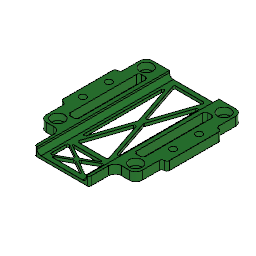
RM Carriage Setup (Goalie) (Autodesk Fusion 360 archive; units mm, degrees)
design "LGR RM Carriage Bracket (Goalie)"
Autodesk Fusion 360 part; units mm, degrees
(part 1 of 2)
sketch "Sketch1" plane through (0, 0, 0) normal (0, 0, 1) x (1, 0, 0)
  line L0 (-41, 41) -> (41, 41)
  line L1 (41, 41) -> (41, -41)
  line L2 (41, -41) -> (-41, -41)
  line L3 (-41, -41) -> (-41, 41)
  dimension "d1" = 82
  dimension "d2" = 82
  dimension "d3" = 41
  dimension "d4" = 41
  constraint horizontal L0
  constraint vertical L1
  constraint horizontal L2
  constraint vertical L3
  measures "d1" distance of L1 L3
  measures "d2" distance of L0 L2
  measures "d3" distance of origin L1
  measures "d4" distance of origin L0
extrude "Extrude1" add sketch "Sketch1" along normal blind 6.5
sketch "Sketch2" plane through (0, 0, 6.5) normal (0, 0, 1) x (-1, 0, 0)
  line L0 (41, 41) -> (-41, 41)
  line L1 (-41, 41) -> (-41, -41)
  line L2 (-41, -41) -> (41, -41)
  line L3 (41, -41) -> (41, 41)
  point P0 (34, -30)
  point P1 (-34, -30)
  point P2 (-34, 30)
  point P3 (34, 30)
  dimension "d7" = 68
  dimension "d8" = 60
  dimension "d9" = 7
  dimension "d10" = 11
  constraint horizontal P0 P1
  constraint vertical P1 P2
  constraint horizontal P2 P3
  constraint vertical P0 P3
  measures "d7" distance of P0 P1
  measures "d8" distance of P1 P2
  measures "d9" distance of L1 P1
  measures "d10" distance of L2 P1
hole "Hole1" at (-34, 30, 6.5) at (34, 30, 6.5) at (34, -30, 6.5) at (-34, -30, 6.5) direction (0, 0, -1) diameter 5.5 depth 10 tip angle 180 counterbore diameter 10 counterbore depth 5
sketch "Sketch3" plane through (0, 0, 6.5) normal (0, 0, 1) x (-1, 0, 0)
  circle A0 centre (-34, 30) radius 5
  circle A1 centre (34, -30) radius 5
  circle A2 centre (-34, -30) radius 5
  circle A3 centre (34, 30) radius 5
  line L0 (41, 41) -> (-41, 41)
  line L1 (-41, 41) -> (-41, -41)
  line L2 (-41, -41) -> (41, -41)
  line L3 (41, -41) -> (41, 41)
  line L4 (41, -19.05) -> (-41, -19.05)
  line L5 (-41, -19.05) -> (-41, 19.05)
  line L6 (-41, 19.05) -> (41, 19.05)
  line L7 (41, 19.05) -> (41, -19.05)
  dimension "d16" = 38.1
  dimension "d17" = 19.05
  constraint horizontal L4
  constraint vertical L5
  constraint horizontal L6
  constraint vertical L7
  constraint coincident L1 L5.end
  constraint coincident L3 L4.start
  measures "d16" distance of L4 L6
  measures "d17" distance of origin L6
extrude "Extrude2" cut sketch "Sketch3" against normal blind 4.5 contours L1 L3 L4 L5 L6 L7
fillet "Fillet1" radius 3 2 edges at (0, 19.05, 2) (0, -19.05, 2)
sketch "Sketch4" plane through (0, 0, 6.5) normal (0, 0, 1) x (-1, 0, 0)
  line L0 (41, -19.05) -> (-41, -19.05)
  line L1 (-41, -19.05) -> (-41, -41)
  line L2 (-41, -41) -> (41, -41)
  line L3 (41, -41) -> (41, -19.05)
  circle A0 centre (34, -30) radius 5
  circle A1 centre (-34, -30) radius 5
  line L4 (41, 41) -> (-41, 41)
  line L5 (41, 19.05) -> (41, 41)
  point P0 (-10, -34.75)
  point P1 (10, -34.75)
  point P2 (-10, 34.75)
  point P3 (10, 34.75)
  point P4 (-5.7919, 53.9874)
  dimension "d23" = 6.25
  dimension "d24" = 6.25
  dimension "d25" = 20
  dimension "d26" = 31
  constraint vertical P0 P2
  constraint horizontal P2 P3
  constraint vertical P1 P3
  constraint horizontal P0 P1
  measures "d23" distance of P2 L4
  measures "d24" distance of L2 P0
  measures "d25" distance of P0 P1
  measures "d26" distance of P3 L5
hole "Hole2" at (10, 34.75, 6.5) at (-10, 34.75, 6.5) at (10, -34.75, 6.5) at (-10, -34.75, 6.5) direction (0, 0, -1) diameter 5 end through all
sketch "Sketch7" plane through (0, 0, 6.5) normal (0, 0, 1) x (-1, 0, 0)
  circle A0 centre (-10, 34.75) radius 2.5
  circle A1 centre (10, 34.75) radius 2.5
  line L0 (-41, 19.05) -> (41, 19.05)
  line L1 (41, 19.05) -> (41, 41)
  line L2 (41, 41) -> (-41, 41)
  line L3 (-41, 41) -> (-41, 19.05)
  circle A2 centre (34, 30) radius 5
  circle A3 centre (-34, 30) radius 5
  line L4 (25.5, 22.05) -> (-25.5, 22.05)
  line L5 (-27.5, 24.05) -> (-27.5, 27.05)
  line L6 (-25.5, 29.05) -> (25.5, 29.05)
  line L7 (27.5, 27.05) -> (27.5, 24.05)
  line L8 (25.5, -29.05) -> (-25.5, -29.05)
  line L9 (-27.5, -27.05) -> (-27.5, -24.05)
  line L10 (-25.5, -22.05) -> (25.5, -22.05)
  line L11 (27.5, -24.05) -> (27.5, -27.05)
  line L12 (41, -19.05) -> (-41, -19.05)
  line L13 (-41, -19.05) -> (-41, -41)
  arc A4 (25.5, -29.05) -> (27.5, -27.05) centre (25.5, -27.05) ccw
  arc A5 (27.5, -24.05) -> (25.5, -22.05) centre (25.5, -24.05) ccw
  arc A6 (-25.5, -22.05) -> (-27.5, -24.05) centre (-25.5, -24.05) ccw
  arc A7 (-27.5, -27.05) -> (-25.5, -29.05) centre (-25.5, -27.05) ccw
  arc A8 (25.5, 22.05) -> (27.5, 24.05) centre (25.5, 24.05) ccw
  arc A9 (27.5, 27.05) -> (25.5, 29.05) centre (25.5, 27.05) ccw
  arc A10 (-25.5, 29.05) -> (-27.5, 27.05) centre (-25.5, 27.05) ccw
  arc A11 (-27.5, 24.05) -> (-25.5, 22.05) centre (-25.5, 24.05) ccw
  dimension "d31" = 55
  dimension "d32" = 7
  dimension "d33" = 3
  dimension "d34" = 13.5
  dimension "d35" = 7
  dimension "d36" = 3
  dimension "d37" = 13.5
  dimension "d38" = 55
  dimension "d39" = 2
  constraint horizontal L4
  constraint vertical L5
  constraint horizontal L6
  constraint vertical L7
  constraint horizontal L8
  constraint vertical L9
  constraint horizontal L10
  constraint vertical L11
  constraint tangent L8 A4
  constraint tangent L11 A4
  constraint tangent L11 A5
  constraint tangent L10 A5
  constraint equal A4 A5
  constraint tangent L10 A6
  constraint tangent L9 A6
  constraint equal A4 A6
  constraint tangent L9 A7
  constraint tangent L8 A7
  constraint equal A4 A7
  constraint tangent L4 A8
  constraint tangent L7 A8
  constraint equal A4 A8
  constraint tangent L7 A9
  constraint tangent L6 A9
  constraint equal A4 A9
  constraint tangent L6 A10
  constraint tangent L5 A10
  constraint equal A4 A10
  constraint tangent L5 A11
  constraint tangent L4 A11
  constraint equal A4 A11
  measures "d31" distance of L5 L7
  measures "d32" distance of L4 L6
  measures "d33" distance of L0 L4
  measures "d34" distance of L1 L7
  measures "d35" distance of L8 L10
  measures "d36" distance of L10 L12
  measures "d37" distance of L9 L13
  measures "d38" distance of L9 L11
  measures "d39" radius of A4
extrude "Extrude3" cut sketch "Sketch7" against normal blind 6.5 contours L4 L5 L6 L7 A8 A9 A10 A11 | L8 L9 L10 L11 A4 A5 A6 A7
ref_plane "WorkPlane1" through (0, 0, 6.5) normal (0, 0, -1) x (-1, 0, 0)
sketch "Sketch9" plane through (0, 0, 6.5) normal (0, 0, -1) x (-1, 0, 0)
  line L0 (41, 41) -> (21, 41)
  line L1 (21, 41) -> (21, 37)
  line L2 (21, 37) -> (41, 37)
  line L3 (41, 37) -> (41, 41)
  line L4 (-21, 41) -> (-41, 41)
  line L5 (-41, 41) -> (-41, 37)
  line L6 (-41, 37) -> (-21, 37)
  line L7 (-21, 37) -> (-21, 41)
  line L8 (41, -37) -> (21, -37)
  line L9 (21, -37) -> (21, -41)
  line L10 (21, -41) -> (41, -41)
  line L11 (41, -41) -> (41, -37)
  line L12 (-41, -41) -> (-21, -41)
  line L13 (-21, -41) -> (-21, -37)
  line L14 (-21, -37) -> (-41, -37)
  line L15 (-41, -37) -> (-41, -41)
  point P0 (41, 41)
  dimension "d59" = 82
  dimension "d60" = 82
  dimension "d61" = 4
  dimension "d62" = 20
  dimension "d63" = 20
  dimension "d64" = 4
  dimension "d65" = 20
  dimension "d66" = 20
  dimension "d67" = 4
  dimension "d68" = 4
  constraint horizontal L0
  constraint vertical L1
  constraint horizontal L2
  constraint vertical L3
  constraint horizontal L4
  constraint vertical L5
  constraint horizontal L6
  constraint vertical L7
  constraint horizontal L8
  constraint vertical L9
  constraint horizontal L10
  constraint vertical L11
  constraint horizontal L12
  constraint vertical L13
  constraint horizontal L14
  constraint vertical L15
  constraint vertical P0 L10.end
  constraint horizontal P0 L4.end
  constraint vertical L4.end L12.start
  constraint horizontal L10.end L12.start
  constraint vertical P0 L0.start
  constraint horizontal L0.end P0
  measures "d59" distance of L3 L5
  measures "d60" distance of L0 L10
  measures "d61" distance of L0 L2
  measures "d62" distance of L1 L3
  measures "d63" distance of L5 L7
  measures "d64" distance of L4 L6
  measures "d65" distance of L13 L15
  measures "d66" distance of L9 L11
  measures "d67" distance of L8 L10
  measures "d68" distance of L12 L14
extrude "Extrude5" cut sketch "Sketch9" along normal blind 6.5
fillet "Fillet2" radius 5 4 edges at (-41, 37, 3.25) (41, 37, 3.25) (41, -37, 3.25) (-41, -37, 3.25)
fillet "Fillet3" radius 2 8 edges at (-21, -41, 3.25) (-21, -37, 3.25) (21, -37, 3.25) (21, -41, 3.25) (21, 37, 3.25) (21, 41, 3.25) (-21, 41, 3.25) (-21, 37, 3.25)
sketch "Sketch10" plane through (0, 0, 2) normal (0, 0, 1) x (-1, 0, 0)
  line L0 (41, 16.05) -> (-41, 16.05)
  line L1 (-41, 16.05) -> (-41, -16.05)
  line L2 (-41, -16.05) -> (41, -16.05)
  line L3 (41, -16.05) -> (41, 16.05)
  line L4 (29.8377, -14) -> (-29.8377, -14)
  line L5 (29.8377, 14) -> (-29.8377, 14)
  line L6 (37.5, -10.6064) -> (37.5, 10.6064)
  line L7 (-37.5, -10.6064) -> (-37.5, 10.6064)
  line L8 (41, -19.05) -> (-41, -19.05)
  line L9 (30.154, 12.0513) -> (0.3162, 2.1054)
  line L10 (-0.3162, 2.1054) -> (-30.154, 12.0513)
  line L11 (-36.1798, 11.5537) -> (-4.8025, 0.9473)
  line L12 (-4.8025, -0.9473) -> (-36.1798, -11.5537)
  line L13 (-30.154, -12.0513) -> (-0.3162, -2.1054)
  line L14 (0.3162, -2.1054) -> (30.154, -12.0513)
  line L15 (36.1798, -11.5537) -> (4.8025, -0.9473)
  line L16 (4.8025, 0.9473) -> (36.1798, 11.5537)
  arc A0 (29.8377, -14) -> (30.154, -12.0513) centre (29.8377, -13) ccw
  arc A1 (0.3162, -2.1054) -> (-0.3162, -2.1054) centre (0, -3.0541) ccw
  arc A2 (-30.154, -12.0513) -> (-29.8377, -14) centre (-29.8377, -13) ccw
  arc A3 (-37.5, -10.6064) -> (-36.1798, -11.5537) centre (-36.5, -10.6064) ccw
  arc A4 (-36.1798, 11.5537) -> (-37.5, 10.6064) centre (-36.5, 10.6064) ccw
  arc A5 (-4.8025, -0.9473) -> (-4.8025, 0.9473) centre (-5.1228, 0) ccw
  arc A6 (-0.3162, 2.1054) -> (0.3162, 2.1054) centre (0, 3.0541) ccw
  arc A7 (-29.8377, 14) -> (-30.154, 12.0513) centre (-29.8377, 13) ccw
  arc A8 (30.154, 12.0513) -> (29.8377, 14) centre (29.8377, 13) ccw
  arc A9 (37.5, 10.6064) -> (36.1798, 11.5537) centre (36.5, 10.6064) ccw
  arc A10 (36.1798, -11.5537) -> (37.5, -10.6064) centre (36.5, -10.6064) ccw
  arc A11 (4.8025, 0.9473) -> (4.8025, -0.9473) centre (5.1228, 0) ccw
  point P0 (36, -14)
  point P1 (-36, -14)
  point P2 (-37.5, -12)
  point P3 (-37.5, 12)
  point P4 (0, -2)
  point P5 (-2, 0)
  point P6 (0, 2)
  point P7 (2, 0)
  dimension "d75" = 72
  dimension "d76" = 24
  dimension "d77" = 5
  dimension "d78" = 7.05
  dimension "d79" = 2.05
  dimension "d80" = 2.05
  dimension "d81" = 3.5
  dimension "d82" = 3.5
  dimension "d83" = 1
  constraint parallel L2 L4
  constraint perpendicular L3 L5
  constraint perpendicular L5 L6
  constraint perpendicular L4 L7
  constraint coincident P0 L4
  constraint coincident P0 L14
  constraint tangent L4 A0
  constraint tangent L14 A0
  constraint tangent L14 A1
  constraint tangent L13 A1
  constraint equal A0 A1
  constraint coincident P1 L13
  constraint coincident P1 L4
  constraint tangent L13 A2
  constraint tangent L4 A2
  constraint equal A0 A2
  constraint coincident P2 L12
  constraint coincident P2 L7
  constraint tangent L12 A3
  constraint tangent L7 A3
  constraint equal A0 A3
  constraint coincident P3 L7
  constraint coincident P3 L11
  constraint tangent L7 A4
  constraint tangent L11 A4
  constraint equal A0 A4
  constraint tangent L11 A5
  constraint tangent L12 A5
  constraint equal A0 A5
  constraint tangent L10 A6
  constraint tangent L9 A6
  constraint equal A0 A6
  constraint tangent L10 A7
  constraint tangent L5 A7
  constraint equal A0 A7
  constraint tangent L5 A8
  constraint tangent L9 A8
  constraint equal A0 A8
  constraint tangent L16 A9
  constraint tangent L6 A9
  constraint equal A0 A9
  constraint tangent L6 A10
  constraint tangent L15 A10
  constraint equal A0 A10
  constraint tangent L15 A11
  constraint tangent L16 A11
  constraint equal A0 A11
  measures "d75" distance of P0 P1
  measures "d76" distance of P2 P3
  measures "d77" distance of L1 P1
  measures "d78" distance of P2 L8
  measures "d79" distance of L2 L4
  measures "d80" distance of L0 L5
  measures "d81" distance of L1 L7
  measures "d82" distance of L3 L6
  measures "d83" radius of A0
extrude "Extrude6" cut sketch "Sketch10" against normal blind 2 contours L4 L13 L14 A0 A1 A2 | L5 L9 L10 A6 A7 A8 | L6 L15 L16 A9 A10 A11 | L7 L11 L12 A3 A4 A5
extrude "Extrude7" add 1 faces at (8.5, 16.6833, 0) along direction (0, 0, -1) blind 0.25
extrude "Extrude8" add 2 faces at (41, 10.6667, -0.0833) (41, 27.6732, 3.691) along direction (1, 0, 0) blind 20
sketch "Sketch12" plane through (0, 0, 6.5) normal (0, 0, 1) x (-1, 0, 0)
  arc A0 (-19, 41) -> (-21, 39) centre (-19, 39) ccw
  arc A1 (-23, 37) -> (-21, 39) centre (-23, 39) ccw
  line L0 (-23, 37) -> (-36, 37)
  arc A2 (-36, 37) -> (-41, 32) centre (-36, 32) ccw
  line L1 (-41, 32) -> (-61, 32)
  line L2 (-61, 32) -> (-61, 19.05)
  line L3 (-61, 19.05) -> (41, 19.05)
  line L4 (41, 19.05) -> (41, 32)
  arc A3 (41, 32) -> (36, 37) centre (36, 32) ccw
  line L5 (36, 37) -> (23, 37)
  arc A4 (21, 39) -> (23, 37) centre (23, 39) ccw
  arc A5 (21, 39) -> (19, 41) centre (19, 39) ccw
  line L6 (19, 41) -> (-19, 41)
  circle A6 centre (-34, 30) radius 5
  circle A7 centre (34, 30) radius 5
  circle A8 centre (10, 34.75) radius 2.5
  circle A9 centre (-10, 34.75) radius 2.5
  line L7 (-27.5, 24.05) -> (-27.5, 27.05)
  arc A10 (-25.5, 29.05) -> (-27.5, 27.05) centre (-25.5, 27.05) ccw
  line L8 (-25.5, 29.05) -> (25.5, 29.05)
  arc A11 (27.5, 27.05) -> (25.5, 29.05) centre (25.5, 27.05) ccw
  line L9 (27.5, 27.05) -> (27.5, 24.05)
  arc A12 (25.5, 22.05) -> (27.5, 24.05) centre (25.5, 24.05) ccw
  line L10 (25.5, 22.05) -> (-25.5, 22.05)
  arc A13 (-27.5, 24.05) -> (-25.5, 22.05) centre (-25.5, 24.05) ccw
  line L11 (-61, 32) -> (-41, 32)
  line L12 (-41, 32) -> (-41, 21.05)
  line L13 (-41, 21.05) -> (-61, 21.05)
  line L14 (-61, 21.05) -> (-61, 32)
  line L15 (-61, -32) -> (-41, -32)
  line L16 (-41, -32) -> (-41, -21.05)
  line L17 (-41, -21.05) -> (-61, -21.05)
  line L18 (-61, -21.05) -> (-61, -32)
  line L19 (41, -19.05) -> (-61, -19.05)
  dimension "d90" = 2
  dimension "d91" = 20
  dimension "d92" = 2
  dimension "d93" = 20
  dimension "d94" = 64
  constraint horizontal L11
  constraint vertical L12
  constraint horizontal L13
  constraint vertical L14
  constraint coincident L1.end L2.start
  constraint horizontal L15
  constraint vertical L16
  constraint horizontal L17
  constraint vertical L18
  constraint vertical L1.end L15.start
  measures "d90" distance of L3 L13
  measures "d91" distance of L12 L14
  measures "d92" distance of L17 L19
  measures "d93" distance of L16 L18
  measures "d94" distance of L11 L15
extrude "Extrude9" cut sketch "Sketch12" against normal blind 7 contours L1 L2 L11 L12 L13 L14 | L15 L16 L17 L18
fillet "Fillet4" radius 5 2 edges at (41, 21.05, 3.125) (41, -21.05, 3.125)
fillet "Fillet5" radius 1.5 2 edges at (61, 21.05, 3.125) (61, -21.05, 3.125)
sketch "Sketch14" plane through (0, 0, 2) normal (0, 0, 1) x (-1, 0, 0)
  line L0 (37.5, 10.6064) -> (37.5, -10.6064)
  arc A0 (36.1798, -11.5537) -> (37.5, -10.6064) centre (36.5, -10.6064) ccw
  line L1 (36.1798, -11.5537) -> (4.8025, -0.9473)
  arc A1 (4.8025, 0.9473) -> (4.8025, -0.9473) centre (5.1228, 0) ccw
  line L2 (4.8025, 0.9473) -> (36.1798, 11.5537)
  arc A2 (37.5, 10.6064) -> (36.1798, 11.5537) centre (36.5, 10.6064) ccw
  line L3 (30.154, 12.0513) -> (0.3162, 2.1054)
  arc A3 (-0.3162, 2.1054) -> (0.3162, 2.1054) centre (0, 3.0541) ccw
  line L4 (-0.3162, 2.1054) -> (-30.154, 12.0513)
  arc A4 (-29.8377, 14) -> (-30.154, 12.0513) centre (-29.8377, 13) ccw
  line L5 (-29.8377, 14) -> (29.8377, 14)
  arc A5 (30.154, 12.0513) -> (29.8377, 14) centre (29.8377, 13) ccw
  line L6 (-30.154, -12.0513) -> (-0.3162, -2.1054)
  arc A6 (0.3162, -2.1054) -> (-0.3162, -2.1054) centre (0, -3.0541) ccw
  line L7 (0.3162, -2.1054) -> (30.154, -12.0513)
  arc A7 (29.8377, -14) -> (30.154, -12.0513) centre (29.8377, -13) ccw
  line L8 (29.8377, -14) -> (-29.8377, -14)
  arc A8 (-30.154, -12.0513) -> (-29.8377, -14) centre (-29.8377, -13) ccw
  line L9 (-4.8025, -0.9473) -> (-36.1798, -11.5537)
  arc A9 (-37.5, -10.6064) -> (-36.1798, -11.5537) centre (-36.5, -10.6064) ccw
  line L10 (-37.5, -10.6064) -> (-37.5, 10.6064)
  arc A10 (-36.1798, 11.5537) -> (-37.5, 10.6064) centre (-36.5, 10.6064) ccw
  line L11 (-36.1798, 11.5537) -> (-4.8025, 0.9473)
  arc A11 (-4.8025, -0.9473) -> (-4.8025, 0.9473) centre (-5.1228, 0) ccw
  line L12 (41, 16.05) -> (-61, 16.05)
  line L13 (-61, 16.05) -> (-61, -16.05)
  line L14 (-61, -16.05) -> (41, -16.05)
  line L15 (41, -16.05) -> (41, 16.05)
  line L16 (-57.5, 10.5218) -> (-57.5, -10.5218)
  line L17 (-41, 10.5218) -> (-41, -10.5218)
  line L18 (-41.94, -10.7593) -> (-47.2368, -0.9503)
  line L19 (-47.2368, 0.9503) -> (-41.94, 10.7593)
  line L20 (-56.56, 10.7593) -> (-51.2632, 0.9503)
  line L21 (-51.2632, -0.9503) -> (-56.56, -10.7593)
  line L22 (-55.0268, 14) -> (-43.4732, 14)
  line L23 (-42.6049, 12.5039) -> (-48.3818, 2.3944)
  line L24 (-50.1182, 2.3944) -> (-55.8951, 12.5039)
  line L25 (-55.8951, -12.5039) -> (-50.1182, -2.3944)
  line L26 (-48.3818, -2.3944) -> (-42.6049, -12.5039)
  line L27 (-43.4732, -14) -> (-55.0268, -14)
  arc A12 (-55.0268, 14) -> (-55.8951, 12.5039) centre (-55.0268, 13) ccw
  arc A13 (-42.6049, 12.5039) -> (-43.4732, 14) centre (-43.4732, 13) ccw
  arc A14 (-55.8951, -12.5039) -> (-55.0268, -14) centre (-55.0268, -13) ccw
  arc A15 (-43.4732, -14) -> (-42.6049, -12.5039) centre (-43.4732, -13) ccw
  arc A16 (-48.3818, -2.3944) -> (-50.1182, -2.3944) centre (-49.25, -2.8906) ccw
  arc A17 (-50.1182, 2.3944) -> (-48.3818, 2.3944) centre (-49.25, 2.8906) ccw
  arc A18 (-41, 10.5218) -> (-41.94, 10.7593) centre (-41.5, 10.5218) ccw
  arc A19 (-41.94, -10.7593) -> (-41, -10.5218) centre (-41.5, -10.5218) ccw
  arc A20 (-57.5, -10.5218) -> (-56.56, -10.7593) centre (-57, -10.5218) ccw
  arc A21 (-51.2632, -0.9503) -> (-51.2632, 0.9503) centre (-53.023, 0) ccw
  arc A22 (-47.2368, 0.9503) -> (-47.2368, -0.9503) centre (-45.477, 0) ccw
  arc A23 (-56.56, 10.7593) -> (-57.5, 10.5218) centre (-57, 10.5218) ccw
  point P0 (-57.5, 12.5)
  point P1 (-57.5, -12.5)
  point P2 (-47.75, 0)
  point P3 (-50.75, 0)
  point P4 (-49.25, 0.875)
  point P5 (-56.75, -14)
  point P6 (-49.25, -0.875)
  point P7 (-41.75, -14)
  dimension "d106" = 3.5
  dimension "d107" = 3.5
  dimension "d108" = 2.05
  dimension "d109" = 2.05
  dimension "d110" = 25
  dimension "d111" = 12.5
  dimension "d112" = 15
  dimension "d113" = 0.75
  dimension "d114" = 3
  dimension "d115" = 1.75
  dimension "d116" = 1.5
  dimension "d117" = 0.875
  dimension "d118" = 8.25
  dimension "d119" = 1
  dimension "d120" = 0.5
  dimension "d121" = 2
  dimension "d122" = 0.5
  constraint vertical L16
  constraint perpendicular L12 L17
  constraint perpendicular L16 L22
  constraint horizontal P2 P3
  constraint vertical P4 P6
  constraint horizontal origin P2
  constraint tangent L24 A12
  constraint tangent L22 A12
  constraint tangent L22 A13
  constraint tangent L23 A13
  constraint equal A12 A13
  constraint coincident P5 L25
  constraint coincident P5 L27
  constraint tangent L25 A14
  constraint tangent L27 A14
  constraint equal A12 A14
  constraint coincident P7 L27
  constraint coincident P7 L26
  constraint tangent L27 A15
  constraint tangent L26 A15
  constraint equal A12 A15
  constraint coincident P6 L26
  constraint coincident P6 L25
  constraint tangent L26 A16
  constraint tangent L25 A16
  constraint equal A12 A16
  constraint coincident P4 L24
  constraint coincident P4 L23
  constraint tangent L24 A17
  constraint tangent L23 A17
  constraint equal A12 A17
  constraint tangent L19 A18
  constraint tangent L17 A18
  constraint tangent L17 A19
  constraint tangent L18 A19
  constraint equal A18 A19
  constraint coincident P1 L21
  constraint coincident P1 L16
  constraint tangent L21 A20
  constraint tangent L16 A20
  constraint equal A18 A20
  constraint coincident P3 L20
  constraint coincident P3 L21
  constraint tangent L20 A21
  constraint tangent L21 A21
  constraint coincident P2 L18
  constraint coincident P2 L19
  constraint tangent L18 A22
  constraint tangent L19 A22
  constraint equal A21 A22
  constraint coincident P0 L16
  constraint coincident P0 L20
  constraint tangent L16 A23
  constraint tangent L20 A23
  measures "d106" distance of L13 L16
  measures "d107" distance of L10 L17
  measures "d108" distance of L12 L22
  measures "d109" distance of L14 L27
  measures "d110" distance of P0 P1
  measures "d111" vertical distance of origin P0
  measures "d112" distance of P5 P7
  measures "d113" horizontal distance of P1 P5
  measures "d114" distance of P2 P3
  measures "d115" distance of P4 P6
  measures "d116" horizontal distance of P3 P4
  measures "d117" vertical distance of P2 P6
  measures "d118" distance of L17 P4
  measures "d119" radius of A12
  measures "d120" radius of A18
  measures "d121" radius of A21
  measures "d122" radius of A23
extrude "Extrude11" cut sketch "Sketch14" against normal blind 3 contours L16 L20 L21 A20 A21 A23 | L17 L18 L19 A18 A19 A22 | L22 L23 L24 A12 A13 A17 | L25 L26 L27 A14 A15 A16
equation "d3 = ( 82 / 2 ) * 1 mm"
equation "d4 = ( 82 / 2 ) * 1 mm"
equation "d9 = ( ( 82 - 68 ) / 2 ) * 1 mm"
equation "d10 = ( ( 82 - 60 ) / 2 ) * 1 mm"
equation "d17 = ( 38.1 / 2 ) * 1 mm"
equation "d26 = ( ( 82 - 20 ) / 2 ) * 1 mm"
equation "d34 = ( ( 82 - 55 ) / 2 ) * 1 mm"
equation "d37 = ( ( 82 - 55 ) / 2 ) * 1 mm"
equation "d77 = ( ( 82 - 72 ) / 2 ) * 1 mm"
equation "d78 = ( ( 38.1 - 24 ) / 2 ) * 1 mm"
equation "d113 = ( ( 16.5 - 15 ) / 2 ) * 1 mm"
equation "d117 = ( 1.75 / 2 ) * 1 mm"
equation "d118 = ( 16.5 / 2 ) * 1 mm"

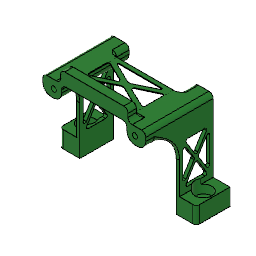
design "LGR RM Front Holder (Goalie)"
Autodesk Fusion 360 part; units mm, degrees
sketch "Sketch1" plane through (0, 0, 0) normal (0, 0, 1) x (1, 0, 0)
  line L0 (28.55, 26.275) -> (30.55, 26.275)
  line L1 (30.55, 26.275) -> (30.55, -26.275)
  line L2 (30.55, -26.275) -> (28.55, -26.275)
  line L3 (28.55, -26.275) -> (28.55, 26.275)
  line L4 (-28.55, -26.275) -> (-30.55, -26.275)
  line L5 (-28.55, 26.275) -> (-28.55, -26.275)
  line L6 (-30.55, -26.275) -> (-30.55, 26.275)
  line L7 (-30.55, 26.275) -> (-28.55, 26.275)
  line L8 (-30.55, 26.275) -> (30.55, 26.275)
  line L9 (30.55, 26.275) -> (30.55, 28.275)
  line L10 (30.55, 28.275) -> (-30.55, 28.275)
  line L11 (-30.55, 28.275) -> (-30.55, 26.275)
  dimension "d1" = 2
  dimension "d2" = 52.55
  dimension "d4" = 26.275
  dimension "d5" = 2
  dimension "d6" = 52.55
  dimension "d7" = 57.1
  dimension "d8" = 28.55
  dimension "d9" = 2
  constraint horizontal L0
  constraint vertical L1
  constraint horizontal L2
  constraint vertical L3
  constraint horizontal L7
  constraint vertical L5
  constraint horizontal L4
  constraint vertical L6
  constraint horizontal L2.end L4.start
  constraint horizontal L8
  constraint vertical L9
  constraint horizontal L10
  constraint vertical L11
  constraint vertical L0.end L9.end
  measures "d1" distance of L1 L3
  measures "d2" distance of L0 L2
  measures "d4" distance of origin L0
  measures "d5" distance of L5 L6
  measures "d6" distance of L4 L7
  measures "d7" distance of L3 L5
  measures "d8" distance of origin L5
  measures "d9" distance of L8 L10
extrude "Extrude1" add sketch "Sketch1" along normal blind 20
sketch "Sketch2" plane through (0, 0, 20) normal (0, 0, 1) x (-1, 0, 0)
  line L0 (-30.55, 26.275) -> (-30.55, -28.275)
  line L1 (-30.55, -28.275) -> (30.55, -28.275)
  line L2 (30.55, -28.275) -> (30.55, 26.275)
  line L3 (30.55, 26.275) -> (28.55, 26.275)
  line L4 (28.55, 26.275) -> (28.55, -26.275)
  line L5 (28.55, -26.275) -> (-28.55, -26.275)
  line L6 (-28.55, -26.275) -> (-28.55, 26.275)
  line L7 (-28.55, 26.275) -> (-30.55, 26.275)
  line L8 (-30.55, 26.275) -> (-40.55, 26.275)
  line L9 (-40.55, 26.275) -> (-40.55, 16.275)
  line L10 (-40.55, 16.275) -> (-30.55, 16.275)
  line L11 (-30.55, 16.275) -> (-30.55, 26.275)
  line L12 (30.55, 26.275) -> (40.55, 26.275)
  line L13 (40.55, 26.275) -> (40.55, 16.275)
  line L14 (40.55, 16.275) -> (30.55, 16.275)
  line L15 (30.55, 16.275) -> (30.55, 26.275)
  dimension "d12" = 10
  dimension "d13" = 10
  dimension "d14" = 10
  dimension "d15" = 10
  constraint horizontal L8
  constraint vertical L9
  constraint horizontal L10
  constraint vertical L11
  constraint coincident L0.start L7.end
  constraint horizontal L12
  constraint vertical L13
  constraint horizontal L14
  constraint vertical L15
  constraint coincident L2.end L3.start
  measures "d12" distance of L8 L10
  measures "d13" distance of L9 L11
  measures "d14" distance of L12 L14
  measures "d15" distance of L13 L15
extrude "Extrude2" add sketch "Sketch2" against normal blind 20 contours L0 L8 L9 L10 L11 | L2 L12 L13 L14 L15
fillet "Fillet1" radius 2 2 edges at (40.55, -21.275, 0) (-40.55, -21.275, 0)
sketch "Sketch3" plane through (0, -16.275, 0) normal (0, 1, 0) x (-1, 0, 0)
  arc A0 (38.55, 0) -> (40.55, 2) centre (38.55, 2) ccw
  line L0 (40.55, 2) -> (40.55, 20)
  line L1 (40.55, 20) -> (30.55, 20)
  line L2 (30.55, 20) -> (30.55, 0)
  line L3 (30.55, 0) -> (38.55, 0)
  point P0 (34.75, 10)
  point P1 (-34.75, 10)
  dimension "d20" = 5.8
  dimension "d21" = 10
  dimension "d22" = 69.5
  constraint horizontal P0 P1
  measures "d20" distance of L0 P0
  measures "d21" distance of L3 P0
  measures "d22" distance of P0 P1
hole "Hole1" at (-34.75, -16.275, 10) at (34.75, -16.275, 10) direction (0, -1, 0) diameter 5.3 end through all counterbore diameter 10 counterbore depth 5
sketch "Sketch4" plane through (0, -16.275, 0) normal (0, 1, 0) x (-1, 0, 0)
  arc A0 (30.55, 7.2871) -> (30.55, 12.7129) centre (34.75, 10) ccw
  line L0 (30.55, 7.2871) -> (30.55, 0)
  line L1 (30.55, 0) -> (38.55, 0)
  arc A1 (38.55, 0) -> (40.55, 2) centre (38.55, 2) ccw
  line L2 (40.55, 2) -> (40.55, 20)
  line L3 (40.55, 20) -> (30.55, 20)
  line L4 (30.55, 20) -> (30.55, 12.7129)
  circle A2 centre (34.75, 10) radius 5
  circle A3 centre (-34.75, 10) radius 5
  dimension "d28" = 10
  dimension "d29" = 69.5
  constraint concentric A0 A2
  constraint coincident A0.end A2
  constraint horizontal A0.centre A3.centre
  measures "d28" diameter of A3
  measures "d29" distance of A0.centre A3.centre
extrude "Extrude3" cut sketch "Sketch4" along normal blind 7 contours A0 A2 | A3
sketch "Sketch5" plane through (0, 28.275, 0) normal (0, 1, 0) x (-1, 0, 0)
  line L0 (-30.55, 0) -> (30.55, 0)
  line L1 (30.55, 0) -> (30.55, 20)
  line L2 (30.55, 20) -> (-30.55, 20)
  line L3 (-30.55, 20) -> (-30.55, 0)
  line L4 (-20, 20) -> (20, 20)
  line L5 (20, 20) -> (20, 0)
  line L6 (20, 0) -> (-20, 0)
  line L7 (-20, 0) -> (-20, 20)
  dimension "d32" = 40
  dimension "d96" = 20
  constraint horizontal L4
  constraint vertical L5
  constraint horizontal L6
  constraint vertical L7
  constraint coincident L0 L5.end
  constraint coincident L2 L4.start
  measures "d32" distance of L5 L7
  measures "d96" distance of origin L7
extrude "Extrude4" add sketch "Sketch5" along normal blind 10 contours L0 L2 L4 L5 L6 L7
sketch "Sketch6" plane through (0, 0, 0) normal (0, 0, -1) x (1, 0, 0)
  line L0 (20, -38.275) -> (20, -28.275)
  line L1 (-30.55, -28.275) -> (-20, -28.275)
  line L2 (30.55, -28.275) -> (30.55, 16.275)
  line L3 (30.55, 16.275) -> (38.55, 16.275)
  line L4 (38.55, 16.275) -> (38.55, 26.275)
  line L5 (38.55, 26.275) -> (28.55, 26.275)
  line L6 (28.55, 26.275) -> (28.55, -26.275)
  line L7 (28.55, -26.275) -> (-28.55, -26.275)
  line L8 (-28.55, -26.275) -> (-28.55, 26.275)
  line L9 (-28.55, 26.275) -> (-38.55, 26.275)
  line L10 (-38.55, 26.275) -> (-38.55, 16.275)
  line L11 (-38.55, 16.275) -> (-30.55, 16.275)
  line L12 (-30.55, 16.275) -> (-30.55, -28.275)
  line L13 (-20, -28.275) -> (-20, -38.275)
  line L14 (-20, -38.275) -> (20, -38.275)
  line L15 (-28.55, -26.275) -> (-19.3, -26.275)
  line L16 (-19.3, -23.775) -> (-19.3, -22.025)
  line L17 (-24.3, -17.025) -> (-26.05, -17.025)
  line L18 (-28.55, -17.025) -> (-28.55, -26.275)
  line L19 (28.55, -26.275) -> (19.3, -26.275)
  line L20 (19.3, -23.775) -> (19.3, -22.025)
  line L21 (24.3, -17.025) -> (26.05, -17.025)
  line L22 (28.55, -17.025) -> (28.55, -26.275)
  arc A0 (-19.3, -22.025) -> (-24.3, -17.025) centre (-24.3, -22.025) ccw
  arc A1 (24.3, -17.025) -> (19.3, -22.025) centre (24.3, -22.025) ccw
  line L23 (28.55, -14.525) -> (28.55, -10)
  line L24 (-28.55, -14.525) -> (-28.55, -10)
  arc A2 (26.05, -17.025) -> (28.55, -14.525) centre (26.05, -14.525) ccw
  arc A3 (-28.55, -14.525) -> (-26.05, -17.025) centre (-26.05, -14.525) ccw
  line L25 (16.8, -26.275) -> (13, -26.275)
  line L26 (-16.8, -26.275) -> (-13, -26.275)
  arc A4 (16.8, -26.275) -> (19.3, -23.775) centre (16.8, -23.775) ccw
  arc A5 (-19.3, -23.775) -> (-16.8, -26.275) centre (-16.8, -23.775) ccw
  line L27 (20, -28.275) -> (30.55, -28.275)
  dimension "d38" = 9.25
  dimension "d39" = 9.25
  dimension "d40" = 9.25
  dimension "d41" = 9.25
  dimension "d42" = 5
  dimension "d43" = 5
  dimension "d44" = 2.5
  dimension "d45" = 2.5
  dimension "d46" = 2.5
  dimension "d47" = 2.5
  constraint horizontal L15
  constraint vertical L16
  constraint horizontal L17
  constraint vertical L18
  constraint coincident L7.end L8.start
  constraint horizontal L19
  constraint vertical L20
  constraint horizontal L21
  constraint vertical L22
  constraint coincident L6.end L7.start
  constraint tangent L17 A0
  constraint tangent L16 A0
  constraint tangent L21 A1
  constraint tangent L20 A1
  constraint coincident L6 L23.end
  constraint coincident L8 L24.end
  constraint coincident L22.start L21
  constraint coincident L22.start L23
  constraint tangent L21 A2
  constraint tangent L23 A2
  constraint coincident L18.start L24
  constraint coincident L18.start L17
  constraint tangent L24 A3
  constraint tangent L17 A3
  constraint coincident L7 L25.end
  constraint coincident L7 L26.end
  constraint coincident L19.end L25
  constraint coincident L19.end L20
  constraint tangent L25 A4
  constraint tangent L20 A4
  constraint coincident L15.end L26
  constraint coincident L15.end L16
  constraint tangent L26 A5
  constraint tangent L16 A5
  measures "d38" distance of L16 L18
  measures "d39" distance of L15 L17
  measures "d40" distance of L20 L22
  measures "d41" distance of L19 L21
  measures "d42" radius of A0
  measures "d43" radius of A1
  measures "d44" radius of A2
  measures "d45" radius of A3
  measures "d46" radius of A4
  measures "d47" radius of A5
extrude "Extrude5" add sketch "Sketch6" against normal blind 20 contours L6 L7 L19 L20 L21 L22 A1 A2 A4 | L7 L8 L15 L16 L17 L18 A0 A3 A5
sketch "Sketch7" plane through (0, 0, 20) normal (0, 0, 1) x (-1, 0, 0)
  line L0 (-30.55, -28.275) -> (-20, -28.275)
  line L1 (-20, -28.275) -> (20, -28.275)
  line L2 (30.55, -28.275) -> (30.55, 16.275)
  line L3 (30.55, 16.275) -> (40.55, 16.275)
  line L4 (40.55, 16.275) -> (40.55, 26.275)
  line L5 (40.55, 26.275) -> (28.55, 26.275)
  line L6 (28.55, 26.275) -> (28.55, -14.525)
  arc A0 (26.05, -17.025) -> (28.55, -14.525) centre (26.05, -14.525) ccw
  line L7 (26.05, -17.025) -> (24.3, -17.025)
  arc A1 (24.3, -17.025) -> (19.3, -22.025) centre (24.3, -22.025) ccw
  line L8 (19.3, -22.025) -> (19.3, -23.775)
  arc A2 (16.8, -26.275) -> (19.3, -23.775) centre (16.8, -23.775) ccw
  line L9 (16.8, -26.275) -> (-16.8, -26.275)
  arc A3 (-19.3, -23.775) -> (-16.8, -26.275) centre (-16.8, -23.775) ccw
  line L10 (-19.3, -23.775) -> (-19.3, -22.025)
  arc A4 (-19.3, -22.025) -> (-24.3, -17.025) centre (-24.3, -22.025) ccw
  line L11 (-24.3, -17.025) -> (-26.05, -17.025)
  arc A5 (-28.55, -14.525) -> (-26.05, -17.025) centre (-26.05, -14.525) ccw
  line L12 (-28.55, -14.525) -> (-28.55, 26.275)
  line L13 (-28.55, 26.275) -> (-40.55, 26.275)
  line L14 (-40.55, 26.275) -> (-40.55, 16.275)
  line L15 (-40.55, 16.275) -> (-30.55, 16.275)
  line L16 (-30.55, 16.275) -> (-30.55, -28.275)
  line L17 (20, -28.275) -> (30.55, -28.275)
  point P0 (24.05, -21.775)
  point P1 (-24.05, -21.775)
  dimension "d52" = 6.5
  dimension "d54" = 6.5
  constraint horizontal P0 P1
  measures "d52" distance of L2 P0
  measures "d54" distance of L16 P1
hole "Hole2" at (-24.05, 21.775, 20) at (24.05, 21.775, 20) direction (0, 0, -1) diameter 3 end through all
sketch "Sketch10" plane through (-30.55, 0, 0) normal (-1, 0, 0) x (0, -1, 0)
  line L0 (-28.275, 0) -> (16.275, 0)
  line L1 (16.275, 0) -> (16.275, 7.2871)
  line L2 (16.275, 7.2871) -> (9.275, 7.2871)
  line L3 (9.275, 7.2871) -> (9.275, 12.7129)
  line L4 (9.275, 12.7129) -> (16.275, 12.7129)
  line L5 (16.275, 12.7129) -> (16.275, 20)
  line L6 (16.275, 20) -> (-28.275, 20)
  line L7 (-11.225, 15.2411) -> (-11.225, 4.8453)
  line L8 (13.275, 15.2453) -> (13.275, 4.8411)
  line L9 (-28.275, 20) -> (-28.275, 0)
  line L10 (-6.5475, 18) -> (8.5844, 18)
  line L11 (-6.5475, 2) -> (8.5844, 2)
  line L12 (-7.0853, 3.8431) -> (0.4635, 8.6578)
  line L13 (1.5372, 8.6589) -> (9.1204, 3.8442)
  line L14 (11.7503, 3.9899) -> (3.3712, 9.1548)
  line L15 (3.3657, 10.854) -> (11.7448, 16.0932)
  line L16 (9.1204, 16.1558) -> (1.5372, 11.3411)
  line L17 (0.4635, 11.3422) -> (-7.0853, 16.1569)
  line L18 (-9.6931, 16.0879) -> (-1.358, 10.8529)
  line L19 (-1.3634, 9.1558) -> (-9.6986, 3.9951)
  arc A0 (-9.6931, 16.0879) -> (-11.225, 15.2411) centre (-10.225, 15.2411) ccw
  arc A1 (-11.225, 4.8453) -> (-9.6986, 3.9951) centre (-10.225, 4.8453) ccw
  arc A2 (-1.3634, 9.1558) -> (-1.358, 10.8529) centre (-1.8898, 10.0061) ccw
  arc A3 (1.5372, 8.6589) -> (0.4635, 8.6578) centre (1.0012, 7.8147) ccw
  arc A4 (8.5844, 2) -> (9.1204, 3.8442) centre (8.5844, 3) ccw
  arc A5 (-7.0853, 3.8431) -> (-6.5475, 2) centre (-6.5475, 3) ccw
  arc A6 (11.7503, 3.9899) -> (13.275, 4.8411) centre (12.275, 4.8411) ccw
  arc A7 (13.275, 15.2453) -> (11.7448, 16.0932) centre (12.275, 15.2453) ccw
  arc A8 (9.1204, 16.1558) -> (8.5844, 18) centre (8.5844, 17) ccw
  arc A9 (-6.5475, 18) -> (-7.0853, 16.1569) centre (-6.5475, 17) ccw
  arc A10 (0.4635, 11.3422) -> (1.5372, 11.3411) centre (1.0012, 12.1853) ccw
  arc A11 (3.3657, 10.854) -> (3.3712, 9.1548) centre (3.8959, 10.0061) ccw
  line L20 (-28.275, 20) -> (-28.275, 0)
  point P0 (-11.225, 17.05)
  point P1 (-11.225, 3.05)
  point P2 (13.275, 17.05)
  point P3 (13.275, 3.05)
  point P4 (-9.975, 18)
  point P5 (12.025, 18)
  point P6 (-9.975, 2)
  point P7 (12.025, 2)
  point P8 (1.025, 10.05)
  point P9 (1, 9)
  point P10 (0, 10)
  point P11 (1, 11)
  point P12 (2, 10)
  dimension "d77" = 3
  dimension "d78" = 17.05
  dimension "d79" = 2
  dimension "d80" = 2
  dimension "d81" = 11
  dimension "d82" = 7
  dimension "d83" = 22
  dimension "d84" = 22
  dimension "d85" = 14
  dimension "d86" = 14
  dimension "d87" = 4.25
  dimension "d88" = 3.05
  dimension "d89" = 1
  constraint perpendicular L6 L7
  constraint vertical L8
  constraint horizontal L10
  constraint perpendicular L7 L11
  constraint horizontal P0 P2
  constraint vertical P4 P6
  constraint coincident P0 L18
  constraint coincident P0 L7
  constraint tangent L18 A0
  constraint tangent L7 A0
  constraint coincident P1 L7
  constraint coincident P1 L19
  constraint tangent L7 A1
  constraint tangent L19 A1
  constraint equal A0 A1
  constraint tangent L19 A2
  constraint tangent L18 A2
  constraint equal A0 A2
  constraint tangent L12 A3
  constraint tangent L13 A3
  constraint equal A0 A3
  constraint coincident P7 L13
  constraint coincident P7 L11
  constraint tangent L13 A4
  constraint tangent L11 A4
  constraint equal A0 A4
  constraint coincident P6 L11
  constraint coincident P6 L12
  constraint tangent L11 A5
  constraint tangent L12 A5
  constraint equal A0 A5
  constraint coincident P3 L14
  constraint coincident P3 L8
  constraint tangent L14 A6
  constraint tangent L8 A6
  constraint equal A0 A6
  constraint coincident P2 L8
  constraint coincident P2 L15
  constraint tangent L8 A7
  constraint tangent L15 A7
  constraint equal A0 A7
  constraint coincident P5 L16
  constraint coincident P5 L10
  constraint tangent L16 A8
  constraint tangent L10 A8
  constraint equal A0 A8
  constraint coincident P4 L17
  constraint coincident P4 L10
  constraint tangent L17 A9
  constraint tangent L10 A9
  constraint equal A0 A9
  constraint tangent L16 A10
  constraint tangent L17 A10
  constraint equal A0 A10
  constraint tangent L14 A11
  constraint tangent L15 A11
  constraint equal A0 A11
  measures "d77" distance of L5 L8
  measures "d78" distance of L7 L9
  measures "d79" distance of L6 L10
  measures "d80" distance of L0 L11
  measures "d81" horizontal distance of P5 P8
  measures "d82" vertical distance of P2 P8
  measures "d83" distance of P4 P5
  measures "d84" distance of P6 P7
  measures "d85" distance of P2 P3
  measures "d86" distance of P0 P1
  measures "d87" distance of L5 P5
  measures "d88" distance of L0 P3
  measures "d89" radius of A0
extrude "Extrude8" cut sketch "Sketch10" against normal blind 65 contours L2 L3 L4 L8 L14 L15 A6 A7 A11 | L2 L3 L4 L8 | L7 L18 L19 A0 A1 A2 | L10 L16 L17 A8 A9 A10 | L11 L12 L13 A3 A4 A5
extrude "Extrude9" cut 2 faces at (27.0333, 28.275, 6.6667) (-23.5167, 28.275, 13.3333) along direction (0, -1, 0) blind 1.55
extrude "Extrude10" cut 1 faces at (-6.6667, 38.275, 13.3333) along direction (0, -1, 0) blind 4.5
fillet "Fillet4" radius 2.5 6 edges at (-20, 26.725, 10) (-20, 33.775, 10) (-30.55, 26.725, 10) (20, 33.775, 10) (20, 26.725, 10) (30.55, 26.725, 10)
sketch "Sketch11" plane through (0, 33.775, 0) normal (0, 1, 0) x (-1, 0, 0)
  line L0 (-17.5, 20) -> (-17.5, 0)
  line L1 (-17.5, 0) -> (17.5, 0)
  line L2 (17.5, 0) -> (17.5, 20)
  line L3 (17.5, 20) -> (-17.5, 20)
  line L4 (-22.5, 4.5) -> (22.5, 4.5)
  line L5 (22.5, 4.5) -> (22.5, 20)
  line L6 (22.5, 20) -> (-22.5, 20)
  line L7 (-22.5, 20) -> (-22.5, 4.5)
  dimension "d99" = 4.5
  dimension "d100" = 45
  dimension "d101" = 15.5
  dimension "d102" = 22.5
  constraint horizontal L4
  constraint vertical L5
  constraint horizontal L6
  constraint vertical L7
  measures "d99" distance of L1 L4
  measures "d100" distance of L5 L7
  measures "d101" distance of L4 L6
  measures "d102" distance of origin L7
extrude "Extrude11" cut sketch "Sketch11" against normal blind 7.05 contours L0 L2 L3 L4 L6 | L0 L4 L6 L7 | L2 L4 L5 L6
fillet "Fillet7" radius 2 1 edges at (0, 26.725, 4.5)
sketch "Sketch15" plane through (0, 26.725, 0) normal (0, 1, 0) x (-1, 0, 0)
  line L0 (-22.5, 0) -> (-22.5, 6.5)
  line L1 (-22.5, 6.5) -> (22.5, 6.5)
  line L2 (22.5, 6.5) -> (22.5, 0)
  line L3 (22.5, 0) -> (28.05, 0)
  line L4 (28.05, 0) -> (28.05, 20)
  line L5 (28.05, 20) -> (-28.05, 20)
  line L6 (-28.05, 20) -> (-28.05, 0)
  line L7 (-28.05, 0) -> (-22.5, 0)
  line L8 (22.5, 6.5) -> (-22.5, 6.5)
  line L9 (-22.5, 6.5) -> (-22.5, 0)
  line L10 (-22.5, 0) -> (22.5, 0)
  line L11 (22.5, 0) -> (22.5, 6.5)
  constraint horizontal L8
  constraint vertical L9
  constraint horizontal L10
  constraint vertical L11
  constraint coincident L0.start L7.end
  constraint coincident L1.end L2.start
extrude "Extrude15" cut sketch "Sketch15" along normal blind 15 contours L0 L1 L2 L8 L9 L10 L11
sketch "Sketch16" plane through (0, 0, 0) normal (0, 0, -1) x (1, 0, 0)
  circle A0 centre (24.05, -21.775) radius 1.5
  circle A1 centre (-24.05, -21.775) radius 1.5
  line L0 (-28.05, -26.725) -> (28.05, -26.725)
  arc A2 (28.05, -26.725) -> (30.55, -24.225) centre (28.05, -24.225) ccw
  line L1 (30.55, -24.225) -> (30.55, 16.275)
  line L2 (30.55, 16.275) -> (38.55, 16.275)
  line L3 (38.55, 16.275) -> (38.55, 26.275)
  line L4 (38.55, 26.275) -> (28.55, 26.275)
  line L5 (28.55, 26.275) -> (28.55, -14.525)
  arc A3 (26.05, -17.025) -> (28.55, -14.525) centre (26.05, -14.525) ccw
  line L6 (26.05, -17.025) -> (24.3, -17.025)
  arc A4 (24.3, -17.025) -> (19.3, -22.025) centre (24.3, -22.025) ccw
  line L7 (19.3, -22.025) -> (19.3, -23.775)
  arc A5 (16.8, -26.275) -> (19.3, -23.775) centre (16.8, -23.775) ccw
  line L8 (16.8, -26.275) -> (-16.8, -26.275)
  arc A6 (-19.3, -23.775) -> (-16.8, -26.275) centre (-16.8, -23.775) ccw
  line L9 (-19.3, -23.775) -> (-19.3, -22.025)
  arc A7 (-19.3, -22.025) -> (-24.3, -17.025) centre (-24.3, -22.025) ccw
  line L10 (-24.3, -17.025) -> (-26.05, -17.025)
  arc A8 (-28.55, -14.525) -> (-26.05, -17.025) centre (-26.05, -14.525) ccw
  line L11 (-28.55, -14.525) -> (-28.55, 26.275)
  line L12 (-28.55, 26.275) -> (-38.55, 26.275)
  line L13 (-38.55, 26.275) -> (-38.55, 16.275)
  line L14 (-38.55, 16.275) -> (-30.55, 16.275)
  line L15 (-30.55, 16.275) -> (-30.55, -24.225)
  arc A9 (-30.55, -24.225) -> (-28.05, -26.725) centre (-28.05, -24.225) ccw
  line L16 (25.55, -17.025) -> (24.3, -17.025)
  line L17 (-30.55, -22.025) -> (-30.55, -24.225)
  line L18 (-28.05, -26.725) -> (28.05, -26.725)
  line L19 (30.55, -24.225) -> (30.55, -22.025)
  line L20 (19.3, -23.775) -> (19.3, -22.025)
  line L21 (-19.3, -23.775) -> (-19.3, -22.025)
  arc A10 (28.05, -26.725) -> (30.55, -24.225) centre (28.05, -24.225) ccw
  arc A11 (-30.55, -24.225) -> (-28.05, -26.725) centre (-28.05, -24.225) ccw
  arc A12 (24.3, -17.025) -> (19.3, -22.025) centre (24.3, -22.025) ccw
  line L22 (-24.3, -17.025) -> (-25.55, -17.025)
  arc A13 (-19.3, -22.025) -> (-24.3, -17.025) centre (-24.3, -22.025) ccw
  line L23 (16.8, -26.275) -> (-16.8, -26.275)
  arc A14 (16.8, -26.275) -> (19.3, -23.775) centre (16.8, -23.775) ccw
  arc A15 (-19.3, -23.775) -> (-16.8, -26.275) centre (-16.8, -23.775) ccw
  circle A16 centre (24.05, -21.775) radius 1.5
  circle A17 centre (-24.05, -21.775) radius 1.5
  arc A18 (-25.55, -17.025) -> (-30.55, -22.025) centre (-25.55, -22.025) ccw
  arc A19 (30.55, -22.025) -> (25.55, -17.025) centre (25.55, -22.025) ccw
  dimension "d168" = 61.1
  dimension "d169" = 9.7
  dimension "d170" = 38.6
  dimension "d171" = 11.25
  dimension "d172" = 2.5
  dimension "d173" = 5
  dimension "d174" = 5
  dimension "d175" = 0.45
  dimension "d176" = 2.5
  dimension "d177" = 2.5
  dimension "d178" = 5
  dimension "d179" = 5
  constraint horizontal L16
  constraint vertical L17
  constraint horizontal L18
  constraint vertical L19
  constraint perpendicular L16 L20
  constraint perpendicular L16 L21
  constraint tangent L19 A10
  constraint tangent L18 A10
  constraint tangent L18 A11
  constraint tangent L17 A11
  constraint equal A10 A11
  constraint tangent L16 A12
  constraint tangent L20 A12
  constraint tangent L21 A13
  constraint tangent L22 A13
  constraint perpendicular L21 L23
  constraint tangent L23 A14
  constraint tangent L20 A14
  constraint tangent L21 A15
  constraint tangent L23 A15
  constraint concentric A0 A16
  constraint concentric A1 A17
  constraint tangent L22 A18
  constraint tangent L17 A18
  constraint tangent L19 A19
  constraint tangent L16 A19
  measures "d168" distance of L17 L19
  measures "d169" distance of L16 L18
  measures "d170" distance of L20 L21
  measures "d171" distance of L19 L20
  measures "d172" radius of A10
  measures "d173" radius of A12
  measures "d174" radius of A13
  measures "d175" distance of L18 L23
  measures "d176" radius of A14
  measures "d177" radius of A15
  measures "d178" radius of A18
  measures "d179" radius of A19
extrude "Extrude16" add sketch "Sketch16" along normal blind 20 contours L0 A2 L1 L6 A4 L7 A5 L8 A6 L9 A7 L10 L15 A9 L16 L17 L18 L19 L20 L21 A10 A11 A12 L22 A13 L23 A14 A15 A18 A19
sketch "Sketch18" plane through (0, 0, 20) normal (0, 0, 1) x (-1, 0, 0)
  line L0 (-28.05, -26.725) -> (28.05, -26.725)
  arc A0 (28.05, -26.725) -> (30.55, -24.225) centre (28.05, -24.225) ccw
  line L1 (30.55, -24.225) -> (30.55, 16.275)
  line L2 (30.55, 16.275) -> (40.55, 16.275)
  line L3 (40.55, 16.275) -> (40.55, 26.275)
  line L4 (40.55, 26.275) -> (28.55, 26.275)
  line L5 (28.55, 26.275) -> (28.55, -14.525)
  arc A1 (26.05, -17.025) -> (28.55, -14.525) centre (26.05, -14.525) ccw
  line L6 (26.05, -17.025) -> (24.3, -17.025)
  arc A2 (24.3, -17.025) -> (19.3, -22.025) centre (24.3, -22.025) ccw
  line L7 (19.3, -22.025) -> (19.3, -23.775)
  arc A3 (16.8, -26.275) -> (19.3, -23.775) centre (16.8, -23.775) ccw
  line L8 (16.8, -26.275) -> (-16.8, -26.275)
  arc A4 (-19.3, -23.775) -> (-16.8, -26.275) centre (-16.8, -23.775) ccw
  line L9 (-19.3, -23.775) -> (-19.3, -22.025)
  arc A5 (-19.3, -22.025) -> (-24.3, -17.025) centre (-24.3, -22.025) ccw
  line L10 (-24.3, -17.025) -> (-26.05, -17.025)
  arc A6 (-28.55, -14.525) -> (-26.05, -17.025) centre (-26.05, -14.525) ccw
  line L11 (-28.55, -14.525) -> (-28.55, 26.275)
  line L12 (-28.55, 26.275) -> (-40.55, 26.275)
  line L13 (-40.55, 26.275) -> (-40.55, 16.275)
  line L14 (-40.55, 16.275) -> (-30.55, 16.275)
  line L15 (-30.55, 16.275) -> (-30.55, -24.225)
  arc A7 (-30.55, -24.225) -> (-28.05, -26.725) centre (-28.05, -24.225) ccw
  circle A8 centre (24.05, -21.775) radius 1.5
  circle A9 centre (-24.05, -21.775) radius 1.5
  line L16 (19.3, -23.775) -> (-19.3, -23.775)
  line L17 (-19.3, -23.775) -> (-19.3, -26.725)
  line L18 (-19.3, -26.725) -> (19.3, -26.725)
  line L19 (19.3, -26.725) -> (19.3, -23.775)
  dimension "d192" = 2.95
  dimension "d193" = 38.6
  constraint horizontal L16
  constraint vertical L17
  constraint horizontal L18
  constraint vertical L19
  constraint coincident L7.end A3.end
  measures "d192" distance of L16 L18
  measures "d193" distance of L17 L19
extrude "Extrude17" cut sketch "Sketch18" against normal blind 10 contours L0 A3 L8 A4 L17 L18 L19
fillet "Fillet8" radius 2.5 2 edges at (-19.3, 26.725, 15) (19.3, 26.725, 15)
fillet "Fillet9" radius 2.5 4 edges at (20.0322, 25.9928, 10) (19.3, 24, 10) (-19.3, 24, 10) (-20.0322, 25.9928, 10)
fillet "Fillet10" radius 15 2 edges at (29.0855, 18.4895, 0) (-29.0855, 18.4895, 0)
sketch "Sketch20" plane through (0, 26.725, 0) normal (0, 1, 0) x (-1, 0, 0)
  line L0 (-21.8, 12.5) -> (-21.8, 20)
  line L1 (-21.8, 20) -> (-28.05, 20)
  line L2 (-28.05, 20) -> (-28.05, -20)
  line L3 (-28.05, -20) -> (28.05, -20)
  line L4 (28.05, -20) -> (28.05, 20)
  line L5 (28.05, 20) -> (21.8, 20)
  line L6 (21.8, 20) -> (21.8, 12.5)
  spline S0 degree 3 poles (17.4699, 10) (17.7885, 10) (18.1326, 10.0486) (18.7976, 10.2365) (19.1187, 10.3749) (19.8306, 10.7581) (20.2629, 11.0723) (21.0731, 11.7716) (21.4536, 12.1536) (21.8, 12.5) knots 1.263831 1.263831 1.263831 1.263831 1.35941 1.35941 1.454989 1.454989 1.601942 1.601942 1.748896 1.748896 1.748896 1.748896
  line L7 (17.4699, 10) -> (-17.4699, 10)
  spline S1 degree 3 poles (-21.8, 12.5) (-21.4536, 12.1536) (-21.0731, 11.7716) (-20.2629, 11.0723) (-19.8306, 10.7581) (-19.1187, 10.3749) (-18.7976, 10.2365) (-18.1326, 10.0486) (-17.7885, 10) (-17.4699, 10) knots 0 0 0 0 0.146954 0.146954 0.293907 0.293907 0.389486 0.389486 0.485065 0.485065 0.485065 0.485065
  line L8 (20, -20) -> (-20, -20)
  line L9 (-20, -20) -> (-20, -15)
  line L10 (-20, -15) -> (20, -15)
  line L11 (20, -15) -> (20, -20)
  dimension "d224" = 5
  dimension "d225" = 40
  dimension "d226" = 20
  constraint horizontal L8
  constraint vertical L9
  constraint horizontal L10
  constraint vertical L11
  constraint coincident L3 L8.start
  measures "d224" distance of L8 L10
  measures "d225" distance of L9 L11
  measures "d226" distance of origin L9
extrude "Extrude19" add sketch "Sketch20" along normal blind 7.05 contours L3 L8 L9 L10 L11
fillet "Fillet11" radius 2.5 2 edges at (-20, 26.725, -17.5) (-20, 33.775, -17.5)
fillet "Fillet11" radius 2.5 2 edges at (20, 33.775, -17.5) (20, 26.725, -17.5)
fillet "Fillet12" radius 2.5 1 edges at (0, 26.725, -15)